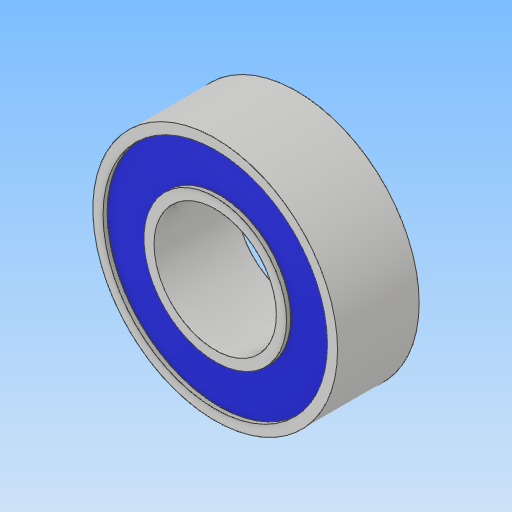
# Autodesk Inventor part: 12x6x4 bearing
Saved by Autodesk Inventor 2020.2 (Build 242310000, 310)
## iProperties
Created: 2018-05-07
Part Number: 12x6x4 bearing
Material: Allgemein
Document SubType Name: Modeling
Designer: paulg
Density: 1 g/cm^3
Appearance: Vorgabe
Author: paulg
Autodesk Inventor part; units mm, degrees
ref_plane "YZ Plane" through (0, 0, 0) normal (1, 0, 0) x (0, 1, 0)
ref_plane "XZ Plane" through (0, 0, 0) normal (0, 1, 0) x (-1, 0, 0)
sketch "Sketch1" plane through (0, 0, 0) normal (0, 0, 1) x (1, 0, 0)
  circle A0 centre (0, 0) radius 6
  circle A1 centre (0, 0) radius 3
  circle A2 centre (0, 0) radius 3.5
  circle A3 centre (0, 0) radius 5.5
  dimension "d0" = 12
  dimension "d1" = 6
  dimension "d2" = 0.5
  dimension "d3" = 0.5
  constraints: 4 centre point, 4 coincident
  measures "d0" diameter of A0
  measures "d1" diameter of A1
  measures "d2" radial gap between concentric circles of A1 A2
  measures "d3" radial gap between concentric circles of A0 A3
extrude "Extrusion1" add sketch "Sketch1" along normal blind 4
ref_plane "Work Plane1" through (0, 0, 0.2) normal (0, 0, 1) x (1, 0, 0)
sketch "Sketch2" plane through (0, 0, 0.2) normal (0, 0, 1) x (1, 0, 0)
  circle A0 centre (0, 0) radius 5.5 projected
  circle A1 centre (0, 0) radius 6 projected
  circle A2 centre (0, 0) radius 3 projected
  circle A3 centre (0, 0) radius 3.5 projected
extrude "Extrusion2" add sketch "Sketch2" along normal blind 3.6 contours A0
body "Solid1"
